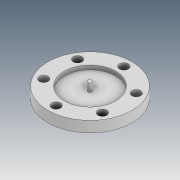
# Autodesk Inventor part: MouldBase
Saved by Autodesk Inventor 2020 (Build 240168000, 168)
## iProperties
Created: 2020-05-07
Part Number: MouldBase
Material: Generic
Document SubType Name: Modeling
Designer: Theo Cominotto
Density: 1 g/cm^3
Appearance: Default
Author: Theo Cominotto
Autodesk Inventor part; units mm, degrees
ref_plane "YZ Plane" through (0, 0, 0) normal (1, 0, 0) x (0, 1, 0)
ref_plane "XZ Plane" through (0, 0, 0) normal (0, 1, 0) x (-1, 0, 0)
ref_plane "XY Plane" through (0, 0, 0) normal (0, 0, 1) x (1, 0, 0)
sketch "Sketch1" plane through (0, 0, 0) normal (0, 0, 1) x (1, 0, 0)
  line L0 (-6.2, 0) -> (37.2, 0) construction
  line L1 (0, -7.2) -> (0, 8.2) construction
  line L2 (1.5, 0) -> (19, 0)
  line L3 (1.5, 0) -> (1.5, 1.5)
  line L4 (19, 0) -> (19, 3)
  line L5 (17, 5) -> (14, 5)
  line L6 (10.5, 1.5) -> (1.5, 1.5)
  line L7 (10.5, 1.5) -> (14, 5)
  line L8 (10.5, 1.5) -> (15.4497, 1.5) construction
  arc A0 (19, 3) -> (17, 5) centre (17, 3) ccw
  line L9 (19, 3) -> (31, 3)
  line L10 (31, 3) -> (31, -5)
  line L11 (31, -5) -> (0, -5)
  line L12 (1.5, 6) -> (0, 6)
  line L13 (0, 6) -> (0, -5)
  line L14 (1.5, 1.5) -> (1.5, 6)
  point P0 (0, 0)
  point P1 (19, 5)
  dimension "d1" = 19
  dimension "d2" = 1.5
  dimension "d3" = 1.5
  dimension "d4" = 5
  dimension "d6" = 45
  dimension "d7" = 10.5
  dimension "d8" = 2
  dimension "d9" = 12
  dimension "d10" = 5
  dimension "d18" = 6
  constraints: 26 end point, 6 point on line, 4 horizontal, 3 perpendicular, 3 vertical, 2 point on circle, 2 tangent, 1 centre point, 1 collinear, 1 equal length
  measures "d1" distance from line of L1 L2.end
  measures "d2" distance from line of L1 L2.start
  measures "d3" distance of L2.start L3.end
  measures "d4" distance of L2.end point (19, 5)
  measures "d6" angle of L8 L7
  measures "d7" distance from line of L1 L6.start
  measures "d8" radius of A0
  measures "d9" distance of L4.end L9.end
  measures "d10" distance between parallel lines of L2 L11
  measures "d18" distance between parallel lines of L0 L12
revolve "Revolution1" add sketch "Sketch1" angle 360 about axis through (0, -10, 0) along (0, 1, 0) contours L2 L4 L9 L10 L11 L13 L12 L14 L3
sketch "Sketch2" plane through (0, -5, 0) normal (0, -1, 0) x (1, 0, 0)
  circle A0 centre (0, 0) radius 31 construction
  circle A1 centre (0, 0) radius 19 construction
  circle A2 centre (0, 0) radius 19 construction
  line L0 (0, 19) -> (0, 31) construction
  circle A3 centre (0, 0) radius 31 construction
  circle A4 centre (0, 25) radius 3.25
  dimension "d12" = 6.5
  constraints: 2 end point, 2 vertical alignment, 1 centre point, 1 midpoint, 1 vertical, 2 other
  measures "d12" diameter of A4
extrude "Extrusion1" cut sketch "Sketch2" against normal up to surface (8 mm away)
pattern_circular "Circular Pattern1" count 6 over 360 about axis through (0, -1, 0) along (0, -1, 0) of "Extrusion1"
body "Solid1"
